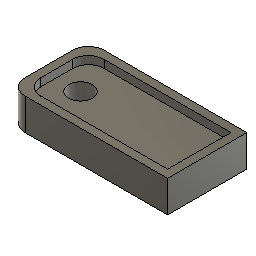
Cube v4 (Autodesk Fusion 360 design; units mm, degrees)
Autodesk Fusion 360 part; units mm, degrees
note: some values were not read from the file. Set by a fixed rule: which sketch regions a step uses.
sketch "Sketch1" plane through (0, 0, 0) normal (0, 1, 0) x (1, 0, 0)
  line L0 (2, 0) -> (20, 0)
  line L1 (20, 0) -> (20, -10)
  line L2 (20, -10) -> (2, -10)
  line L3 (0, -8) -> (0, -2)
  arc A0 (2, 0) -> (0, -2) centre (2, -2) ccw
  arc A1 (0, -8) -> (2, -10) centre (2, -8) ccw
  point P0 (0, -10)
  dimension "d1" = 10
  dimension "d2" = 20
  dimension "d12" = 2
  constraint horizontal L0
  constraint vertical L1
  constraint horizontal L2
  constraint vertical L3
  constraint tangent L0 A0
  constraint tangent L3 A0
  constraint coincident P0 L2
  constraint coincident P0 L3
  constraint tangent L2 A1
  constraint tangent L3 A1
  constraint equal A0 A1
  measures "d1" distance of L0.end L1.end
  measures "d2" distance of L1.end P0
  measures "d12" radius of A0
extrude "Extrude1" add sketch "Sketch1" along normal blind 3
sketch "Sketch2" plane through (0, 3, 0) normal (0, 1, 0) x (-1, 0, 0)
  line L0 (-2, 10) -> (-20, 10)
  line L1 (-20, 10) -> (-20, 0)
  line L2 (-20, 0) -> (-2, 0)
  line L3 (0, 2) -> (0, 8)
  line L4 (-3, 9) -> (-19, 9)
  line L5 (-19, 9) -> (-19, 1)
  line L6 (-19, 1) -> (-3, 1)
  line L7 (-1, 3) -> (-1, 7)
  circle A0 centre (-4, 5) radius 1.5
  line L8 (0, 5) -> (-20, 5) construction
  line L9 (-11, 0) -> (-11, 10) construction
  arc A1 (-2, 0) -> (0, 2) centre (-2, 2) ccw
  arc A2 (0, 8) -> (-2, 10) centre (-2, 8) ccw
  arc A3 (-3, 1) -> (-1, 3) centre (-3, 3) ccw
  arc A4 (-1, 7) -> (-3, 9) centre (-3, 7) ccw
  dimension "d6" = 3
  dimension "d7" = 3
  dimension "d13" = 2
  dimension "d14" = 2
  constraint midpoint L3 L8.start
  constraint midpoint L1 L8.end
  constraint midpoint L2 L9.start
  constraint midpoint L0 L9.end
  constraint coincident A0.centre L8
  constraint parallel L0 L4
  constraint parallel L1 L5
  constraint parallel L2 L6
  constraint parallel L3 L7
  constraint tangent L6 A3
  constraint tangent L7 A3
  constraint tangent L4 A4
  constraint tangent L7 A4
  measures "d6" diameter of A0
  measures "d7" distance of L7 A0.centre
  measures "d13" radius of A3
  measures "d14" radius of A4
extrude "Extrude2" add sketch "Sketch2" along normal blind 1 contours L0 L1 L2 L3 A1 A2
extrude "Extrude3" cut sketch "Sketch2" against normal blind 3 contours A0
